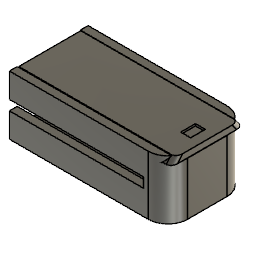
box_cover_wiring (Autodesk Fusion 360 design; units mm, degrees)
Autodesk Fusion 360 part; units mm, degrees
sketch "Sketch1" plane through (0, 0, 0) normal (0, 1, 0) x (1, 0, 0) in component "box"
  line L0 (-11, -75) -> (150, -75)
  line L1 (150, -75) -> (150, -15)
  line L2 (150, -15) -> (-11, -15)
  line L3 (-11, -15) -> (-11, -75)
  dimension "d1_1" = 60
  dimension "d2_1" = 161
  constraint horizontal L0
  constraint vertical L1
  constraint horizontal L2
  constraint vertical L3
  measures "d1_1" distance of L0 L2
  measures "d2_1" distance of L1 L3
extrude "Extrude1" add sketch "Sketch1" along normal blind 80 makes body 1 in component "box"
shell "Shell1" thickness 8 removed faces 2 at (42.6667, 53.3333, 75) at (-11, 26.6667, 35) on bodies 1 in component "box"
sketch "Sketch3" plane through (150, 0, 0) normal (1, 0, 0) x (0, 1, 0) in component "box"
  line L0 (0, 75) -> (0, 15)
  line L1 (0, 15) -> (80, 15)
  line L2 (80, 15) -> (80, 75)
  line L3 (80, 75) -> (0, 75)
  line L4 (8, 75) -> (2.9447, 68.7997)
  line L5 (40, 75) -> (40, 68.7997) construction
  line L6 (40, 68.7997) -> (2.9447, 68.7997)
  line L7 (72, 75) -> (77.0553, 68.7997)
  line L8 (40, 68.7997) -> (77.0553, 68.7997)
  point P0 (8, 75)
  point P1 (72, 75)
  dimension "d13_1" = 8
  constraint coincident P0 L4.start
  constraint midpoint L3 L5.start
  constraint perpendicular L3 L5
  constraint horizontal L4.end L5.end
  constraint symmetric P0 L5 P1
  constraint symmetric L4.end L5 L7.end
  constraint symmetric L6.start L5 L8.start
  measures "d13_1" distance of P0 L4.end
extrude "Extrude3" cut sketch "Sketch3" against normal blind 200 contours L3 L4 L6 L7 L8 bodies 1 in component "box"
fillet "Fillet3" radius 20 1 edges at (150, 0, 45) on bodies 1 in component "box"
fillet "Fillet4" radius 20 1 edges at (150, 80, 45) on bodies 1 in component "box"
sketch "Sketch1 (2)" plane through (-86.6627, 0, 0) normal (-1, 0, 0) x (0, -1, 0)
  line L0 (4.4676, 66.1951) -> (4.4676, 6.1951)
  line L1 (4.4676, 6.1951) -> (84.4676, 6.1951)
  line L2 (84.4676, 6.1951) -> (84.4676, 66.1951)
  line L3 (76.4676, 14.1951) -> (12.4676, 14.1951)
  line L4 (12.4676, 14.1951) -> (12.4676, 59.9948)
  circle A0 centre (80, -30) radius 1.5
  circle A1 centre (-120, -30) radius 1.5
  line L5 (81.5228, 59.9948) -> (76.4676, 59.9948)
  line L6 (7.4123, 59.9948) -> (12.4676, 66.1951)
  line L7 (12.4676, 66.1951) -> (4.4676, 66.1951)
  line L8 (76.4676, 59.9948) -> (76.4676, 14.1951)
  line L9 (84.4676, 66.1951) -> (76.4676, 66.1951)
  line L10 (76.4676, 66.1951) -> (81.5228, 59.9948)
  line L11 (12.4676, 59.9948) -> (7.4123, 59.9948)
  dimension "d1" = 3
  dimension "d2" = 3
  measures "d1" diameter of A0
  measures "d2" diameter of A1
sketch "Sketch2" plane through (0, -48.0314, 0) normal (0, -1, 0) x (1, 0, 0)
  line L0 (54.9401, 42.0285) -> (54.9401, 102.0285)
  line L1 (54.9401, 102.0285) -> (-86.0599, 102.0285)
  line L2 (-86.0599, 102.0285) -> (-86.0599, 42.0285)
  line L3 (-86.0599, 42.0285) -> (54.9401, 42.0285)
  line L4 (54.9401, 72.0285) -> (-86.0599, 72.0285) construction
  line L5 (50.1688, 72.0285) -> (50.1688, 67.0285)
  line L6 (50.1688, 72.0285) -> (50.1688, 77.0285)
  line L7 (50.1688, 77.0285) -> (-86.0599, 77.0285)
  line L8 (50.1688, 67.0285) -> (-86.0599, 67.0285)
  dimension "d5" = 5
  dimension "d6" = 5
  constraint midpoint L0 L4.start
  constraint midpoint L2 L4.end
  constraint coincident L4 L5.start
  constraint perpendicular L4 L5
  constraint perpendicular L4 L6
  constraint coincident L2 L7.end
  constraint perpendicular L2 L7
  constraint coincident L2 L8.end
  constraint perpendicular L2 L8
  measures "d5" distance of L5.start L5.end
  measures "d6" distance of L5.start L6.end
extrude "Extrude8" cut sketch "Sketch2" against normal blind 30 contours L2 L5 L6 L7 L8 sketch seen with x (1, 0, 0) y (0, 1, 0) z (0, 0, 1) at (75.0599, 48.0314, -27.0285) bodies 1 in component "box"
sketch "Sketch3 (2)" plane through (0, 31.9686, 0) normal (0, 1, 0) x (-1, 0, 0)
  line L0 (-54.9401, 102.0285) -> (-54.9401, 42.0285)
  line L1 (-54.9401, 42.0285) -> (86.0599, 42.0285)
  line L2 (86.0599, 42.0285) -> (86.0599, 102.0285)
  line L3 (86.0599, 102.0285) -> (-54.9401, 102.0285)
  line L4 (67.5, 90.4008) -> (86.0599, 90.4008)
  line L5 (86.0599, 90.4008) -> (86.0599, 77.7208)
  line L6 (86.0599, 77.7208) -> (67.5, 77.7208)
  line L7 (65, 80.2208) -> (65, 87.9008)
  arc A0 (67.5, 90.4008) -> (65, 87.9008) centre (67.5, 87.9008) ccw
  arc A1 (65, 80.2208) -> (67.5, 77.7208) centre (67.5, 80.2208) ccw
  dimension "d9" = 2.5
  constraint horizontal L4
  constraint vertical L5
  constraint horizontal L6
  constraint vertical L7
  constraint coincident L2 L5.end
  constraint tangent L4 A0
  constraint tangent L7 A0
  constraint tangent L6 A1
  constraint tangent L7 A1
  constraint equal A0 A1
  measures "d9" radius of A0
extrude "Extrude9" cut sketch "Sketch3 (2)" against normal blind 20 contours L2 L4 L5 L6 L7 A0 A1 sketch seen with x (1, 0, 0) y (0, 1, 0) z (0, 0, 1) at (75.0599, 48.0314, -27.0285) bodies 1 in component "box"
sketch "Sketch1 (3)" plane through (74.9401, 0, 0) normal (1, 0, 0) x (0, 1, 0) in component "lid"
  line L0 (11.9686, 42.0285) -> (11.9686, 95.8282)
  line L1 (11.9686, 95.8282) -> (-28.0314, 95.8282)
  line L2 (-28.0314, 95.8282) -> (-28.0314, 42.0285)
  line L3 (-28.0314, 42.0285) -> (11.9686, 42.0285)
  line L4 (-48.0314, 102.0285) -> (-40.0314, 102.0285)
  line L5 (-40.0314, 102.0285) -> (-45.0867, 95.8282)
  line L6 (-45.0867, 95.8282) -> (-28.0314, 95.8282)
  line L7 (11.9686, 95.8282) -> (-28.0314, 95.8282)
  line L8 (11.9686, 95.8282) -> (29.0239, 95.8282)
  line L9 (29.0239, 95.8282) -> (23.9686, 102.0285)
  line L10 (23.9686, 102.0285) -> (31.9686, 102.0285)
  line L11 (-48.0314, 102.2785) -> (-39.505, 102.2785)
  line L12 (-39.505, 102.2785) -> (-44.5603, 96.0782)
  line L13 (-44.5603, 96.0782) -> (-28.0314, 96.0782)
  line L14 (11.9686, 96.0782) -> (-28.0314, 96.0782)
  line L15 (11.9686, 96.0782) -> (28.4975, 96.0782)
  line L16 (28.4975, 96.0782) -> (23.4422, 102.2785)
  line L17 (23.4422, 102.2785) -> (31.9686, 102.2785)
  line L18 (23.4422, 102.2785) -> (-39.505, 102.2785)
  dimension "d12" = -0.25
  constraint parallel L11 L18
extrude "Extrude1'" add sketch "Sketch1 (3)" against normal blind 160 separate body contours L12 L13 L14 L15 L16 L18 makes body 2 in component "lid"
fillet "Fillet1" radius 5 1 edges at (74.9401, -42.0326, 99.1784) on bodies 2 in component "lid"
fillet "Fillet2" radius 5 1 edges at (74.9401, 25.9698, 99.1784) on bodies 2 in component "lid"
sketch "Sketch2 (2)" plane through (0, 0, 102.2785) normal (0, 0, 1) x (-1, 0, 0) in component "lid"
  ellipse E0 centre (-69.9401, -16.991) end of major axis (-69.9401, -23.4422) minor radius 5 (-74.9401, -16.991) -> (-69.9401, -23.4422) ccw
  line L0 (-69.9401, -23.4422) -> (85.0599, -23.4422)
  line L1 (85.0599, -23.4422) -> (85.0599, 39.505)
  line L2 (85.0599, 39.505) -> (-69.9401, 39.505)
  ellipse E1 centre (-69.9401, 33.0538) end of major axis (-69.9401, 39.505) minor radius 5 (-69.9401, 39.505) -> (-74.9401, 33.0538) ccw
  line L3 (-74.9401, 33.0538) -> (-74.9401, -16.991)
  line L4 (-65, 14.9834) -> (-55, 14.9834)
  line L5 (-55, 14.9834) -> (-55, 0.0818)
  line L6 (-55, 0.0818) -> (-65, 0.0818)
  line L7 (-65, 0.0818) -> (-65, 14.9834)
  constraint horizontal L4
  constraint vertical L5
  constraint horizontal L6
  constraint vertical L7
extrude "Extrude2" cut sketch "Sketch2 (2)" against normal blind 2 contours L4 L5 L6 L7 bodies 2 in component "lid"
component "box" placed x (1, 0, 0) y (0, 1, 0) z (0, 0, 1) at (-75.0599, -48.0314, 27.0285)
component "lid" placed x (1, 0, 0) y (0, 1, 0) z (0, 0, 1) at (0, 0, 0)
